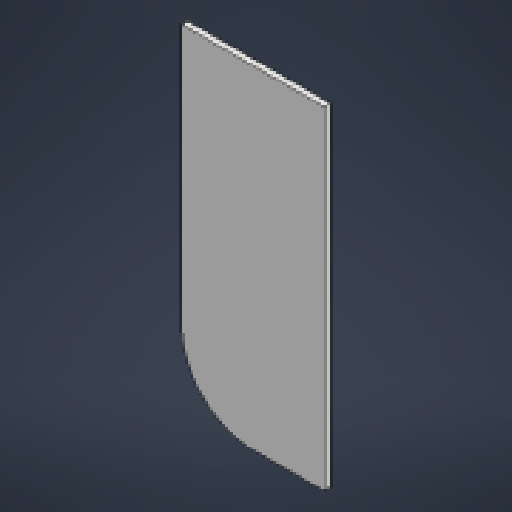
# Autodesk Inventor part: Flywheel base front polycarb
Saved by Autodesk Inventor 2023.2 (Build 272271030, 271C)
## iProperties
Created: 2023-04-01
Part Number: Flywheel base front polycarb
Material: Generic
Document SubType Name: Modeling
Designer: Main Account
Density: 1 g/cm^3
Appearance: Default
Author: Main Account
Autodesk Inventor part; units mm, degrees
ref_plane "YZ Plane" through (0, 0, 0) normal (1, 0, 0) x (0, 1, 0)
ref_plane "XZ Plane" through (0, 0, 0) normal (0, 1, 0) x (-1, 0, 0)
ref_plane "XY Plane" through (0, 0, 0) normal (0, 0, 1) x (1, 0, 0)
sketch "Sketch1" plane through (0, 0, 0) normal (0, 0, 1) x (1, 0, 0)
  line L0 (-5.3154, 38.1) -> (3.9874, 38.1) construction
  line L1 (3.9874, -24.2345) -> (3.9874, 38.1) construction
  line L2 (3.9874, 38.1) -> (-34.1126, 38.1)
  line L3 (-34.1126, 38.1) -> (-34.1126, -31.75)
  line L4 (-15.0626, -50.8) -> (3.9874, -50.8)
  line L5 (3.9874, -50.8) -> (3.9874, 38.1)
  arc A0 (-34.1126, -31.75) -> (-15.0626, -50.8) centre (-15.0626, -31.75) ccw
  point P0 (0, 0)
  point P1 (-34.1126, -50.8)
  dimension "d0" = 38.1
  dimension "d1" = 88.9
  dimension "d2" = 19.05
  constraints: 12 end point, 2 point on circle, 2 point on line, 2 tangent, 1 centre point
  measures "d0" distance of L4.end point (-34.113, -50.8)
  measures "d1" distance of point (-34.113, -50.8) L2.end
  measures "d2" radius of A0
extrude "Extrusion1" add sketch "Sketch1" along normal blind 1.5875
body "Solid1"
